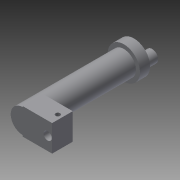
# Autodesk Inventor part: ось
Saved by Autodesk Inventor 2013 (Build 170138000, 138)
## iProperties
Created: 2014-04-30
Part Number: ось
Material: Типовые
Document SubType Name: Modeling
Designer: HP1
Density: 1 g/cm^3
Mass: 7.99008 g
Surface Area: 33.0141 cm^2
Volume: 7.99008 cm^3
Author: HP1
Autodesk Inventor part; units mm, degrees
ref_plane "YZ Plane" through (0, 0, 0) normal (1, 0, 0) x (0, 1, 0)
ref_plane "XZ Plane" through (0, 0, 0) normal (0, 1, 0) x (-1, 0, 0)
ref_plane "XY Plane" through (0, 0, 0) normal (0, 0, 1) x (1, 0, 0)
sketch "Эскиз1" plane through (0, 0, 0) normal (0, 1, 0) x (-1, 0, 0)
  circle A0 centre (0, 0) radius 6
  dimension "d0" = 12
  constraints: 1 centre point
  measures "d0" diameter of A0
extrude "Выдавливание1" add sketch "Эскиз1" along normal blind 50
sketch "Эскиз2" plane through (0, 50, 0) normal (0, 1, 0) x (1, 0, 0)
  circle A0 centre (0, 0) radius 8
  dimension "d3" = 16
  constraints: 1 centre point
  measures "d3" diameter of A0
extrude "Выдавливание2" add sketch "Эскиз2" along normal blind 5
sketch "Эскиз3" plane through (0, 55, 0) normal (0, 1, 0) x (1, 0, 0)
  circle A0 centre (0, 0) radius 8 projected
  circle A1 centre (4, 0) radius 3
  dimension "d6" = 6
  dimension "d7" = 4
  constraints: 1 centre point
  measures "d6" diameter of A1
  measures "d7" distance of A1.centre A0.centre
extrude "Выдавливание3" add sketch "Эскиз3" along normal blind 5 contours A1
sketch "Эскиз4" plane through (0, 0, 0) normal (1, 0, 0) x (0, 1, 0)
  line L0 (0, 6.4352) -> (10.2146, 6.4352)
  line L1 (10.2146, 6.4352) -> (10.2146, -6.6395)
  line L2 (10.2146, -6.6395) -> (0, -6.6395)
  line L3 (0, -6.6395) -> (0, 6.4352)
  point P0 (0, 0)
  constraints: 8 end point, 2 parallel, 1 horizontal, 1 perpendicular
extrude "Выдавливание4" add sketch "Эскиз4" along normal blind 14.5
sketch "Эскиз7" plane through (0, 0, 0) normal (0, -1, 0) x (1, 0, 0)
  circle A0 centre (12.2744, -0.1021) radius 2.0418
  constraints: 1 centre point
extrude "Выдавливание7" cut sketch "Эскиз7" against normal blind 14.5
sketch "Эскиз8" plane through (0, 0, -6.6395) normal (0, 0, -1) x (-1, 0, 0)
  circle A0 centre (-12.2507, 5.1073) radius 1.129
  constraints: 1 centre point
extrude "Выдавливание8" cut sketch "Эскиз8" against normal blind 14.5
